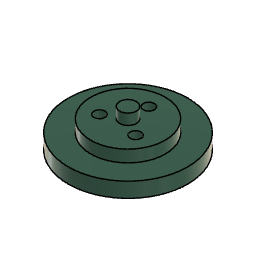
Tapa de rodamiento pata superior (Autodesk Fusion 360 design; units mm, degrees)
Autodesk Fusion 360 part; units mm, degrees
note: some values were not read from the file. Set by a fixed rule: which sketch regions a step uses.
sketch "Boceto9" plane through (0, 0, 0) normal (0, 0, 1) x (1, 0, 0)
  circle A0 centre (0, 0) radius 15
  dimension "d28" = 30
  constraint coincident A0.centre origin
  measures "d28" diameter of A0
extrude "Extruir9" add sketch "Boceto9" along normal blind 4
sketch "Boceto10" plane through (0, 0, 4) normal (0, 0, 1) x (-1, 0, 0)
  circle A0 centre (0, 0) radius 15
  circle A1 centre (0, 0) radius 12.5
  dimension "d31" = 25
  constraint coincident A0.centre A1.centre
  measures "d31" diameter of A1
extrude "Extruir10" add sketch "Boceto10" along normal blind 4 contours A1
sketch "Boceto11" plane through (0, 0, 0) normal (0, 0, -1) x (1, 0, 0)
  circle A0 centre (0, 0) radius 15
  circle A1 centre (0, 0) radius 12.5
  circle A2 centre (0, 0) radius 7
  line L0 (0, 0) -> (-6.0622, 3.5)
  line L1 (0, 0) -> (7, 0) construction
  line L2 (0, 0) -> (6.0622, 3.5)
  line L3 (0, 0) -> (7, 0) construction
  line L4 (0, 0) -> (0, -7)
  circle A3 centre (6.0622, 3.5) radius 3.75
  circle A4 centre (-6.0622, 3.5) radius 3.75
  circle A5 centre (0, -7) radius 3.75
  circle A6 centre (6.0622, 3.5) radius 2
  circle A7 centre (-6.0622, 3.5) radius 2
  circle A8 centre (0, -7) radius 2
  dimension "d34" = 25
  dimension "d35" = 14
  dimension "d36" = 150
  dimension "d37" = 30
  dimension "d38" = 7
  dimension "d39" = 7.5
  dimension "d40" = 7.5
  dimension "d41" = 7.5
  dimension "d42" = 4
  dimension "d43" = 4
  dimension "d44" = 4
  constraint coincident A0.centre A1.centre
  constraint horizontal L1
  constraint horizontal L3
  constraint coincident A2 L4.end
  constraint perpendicular L3 L4
  constraint coincident L2.end A3.centre
  constraint coincident L0.end A4.centre
  constraint coincident L4.end A5.centre
  constraint concentric A3 A6
  constraint concentric A4 A7
  constraint concentric A5 A8
  measures "d34" diameter of A1
  measures "d35" diameter of A2
  measures "d36" angle of L0 L1
  measures "d37" angle of L2 L3
  measures "d38" distance of A0.centre L2.end
  measures "d39" diameter of A3
  measures "d40" diameter of A4
  measures "d41" diameter of A5
  measures "d42" diameter of A6
  measures "d43" diameter of A7
  measures "d44" diameter of A8
extrude "Extruir11" cut sketch "Boceto11" against normal blind 3 contours A2 L2 A3 A6 | A2 A3 A6 | A2 L2 A6 | A2 A6 | A2 L2 A6 | A2 L2 A3 A6 | A2 A5 A8 | A2 L4 A5 A8 | A2 A8 | A2 L4 A8 | A2 L4 A5 A8 | A2 L4 A8 | A2 L0 A4 A7 | A2 L0 A4 A7 | A2 A4 A7 | A2 L0 A7 | A2 L0 A7 | A2 A7
extrude "Extruir12" add 1 faces at (-0.3737, -9.0198, 0) along direction (0, 0, -1) blind 1
extrude "Extruir13" cut sketch "Boceto11" against normal blind 20 contours A2 L2 A6 | A2 A6 | A2 L2 A6 | A2 A8 | A2 L4 A8 | A2 L4 A8 | A2 L0 A7 | A2 L0 A7 | A2 A7
sketch "Boceto12" plane through (0, 0, 8) normal (0, 0, 1) x (-1, 0, 0)
  circle A0 centre (-6.0622, 3.5) radius 2
  circle A1 centre (6.0622, 3.5) radius 2
  circle A2 centre (0, -7) radius 2
  circle A3 centre (0, 0) radius 12.5
  circle A4 centre (0, 0) radius 2.8
  dimension "d51" = 5.6
  constraint coincident A3.centre A4.centre
  measures "d51" diameter of A4
extrude "Extruir14" add sketch "Boceto12" along normal blind 3.6 contours A4
move_face "CarasDesfase2" offset 0.15 3 faces at (-4.0721, -3.3009, 4.6667) (8.0522, -3.3009, 4.6667) (1.9901, 7.1991, 4.6667)
move_face "CarasDesfase3" offset 3 1 faces at (14.9814, -0.7477, 0.6667)
move_face "CarasDesfase4" offset 2 1 faces at (17.9776, -0.8972, 0.6667)
